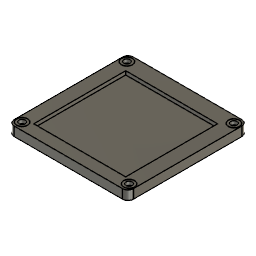
Hub_PCB_TopAndBottomCase_Assembled (Autodesk Fusion 360 archive; units mm, degrees)
design "case"
part number: 2026-03-31-19-00-49-928
Autodesk Fusion 360 part; units mm, degrees
sketch "Sketch1" plane through (0, 0, 0) normal (0, 1, 0) x (1, 0, 0)
  line L0 (0, 0) -> (50, 0)
  line L1 (50, 0) -> (50, 50)
  line L2 (50, 50) -> (0, 50)
  line L3 (0, 50) -> (0, 0)
  line L4 (-7.3367, -6.3969) -> (57.6633, -6.3969)
  line L5 (57.6633, -6.3969) -> (57.6633, 58.6031)
  line L6 (57.6633, 58.6031) -> (-7.3367, 58.6031)
  line L7 (-7.3367, 58.6031) -> (-7.3367, -6.3969)
  circle A0 centre (-3.9367, -2.3969) radius 1.7
  circle A1 centre (54.2633, -2.3969) radius 1.7
  circle A2 centre (54.2633, 54.6031) radius 1.7
  circle A3 centre (-3.9367, 54.6031) radius 1.7
  circle A4 centre (54.2633, 54.6031) radius 3
  circle A5 centre (-3.9367, 54.6031) radius 3
  circle A6 centre (-3.9367, -2.3969) radius 3
  circle A7 centre (54.2633, -2.3969) radius 3
  dimension "d3" = 65
  dimension "d4" = 65
  dimension "d5" = 3.4
  dimension "d6" = 4
  dimension "d7" = 3.4
  dimension "d8" = 3.4
  dimension "d9" = 4
  dimension "d10" = 3.4
  dimension "d11" = 3.4
  dimension "d12" = 3.4
  dimension "d13" = 4
  dimension "d14" = 3.4
  dimension "d15" = 3.4
  dimension "d16" = 4
  dimension "d17" = 6
  dimension "d18" = 6
  dimension "d19" = 6
  dimension "d20" = 6
  constraint horizontal L0
  constraint vertical L1
  constraint horizontal L2
  constraint vertical L3
  constraint coincident L0.start L3.end
  constraint horizontal L4
  constraint vertical L5
  constraint horizontal L6
  constraint vertical L7
  constraint concentric A2 A4
  constraint concentric A3 A5
  constraint concentric A0 A6
  constraint concentric A1 A7
  measures "d3" distance of L4.start L6.end
  measures "d4" distance of L5.end L6.end
  measures "d5" diameter of A0
  measures "d6" distance of L4 A0.centre
  measures "d7" distance of L7 A0.centre
  measures "d8" diameter of A1
  measures "d9" distance of L4 A1.centre
  measures "d10" distance of L5 A1.centre
  measures "d11" diameter of A2
  measures "d12" distance of L5 A2.centre
  measures "d13" distance of L6 A2.centre
  measures "d14" diameter of A3
  measures "d15" distance of L7 A3.centre
  measures "d16" distance of L6 A3.centre
  measures "d17" diameter of A4
  measures "d18" diameter of A5
  measures "d19" diameter of A6
  measures "d20" diameter of A7
extrude "Extrude1" add sketch "Sketch1" along normal blind 2 from surface at 3.1 contours A4 | A5 | A6 | A7 makes body 1 at (-0.9516, 4.4333, -54.3044) makes body 2 at (-0.9516, 4.4333, 2.6956) makes body 3 at (57.2484, 4.4333, -54.3044) makes body 4 at (57.2484, 4.4333, 2.6956)
extrude "Extrude2" add sketch "Sketch1" along normal blind 5 contours L4 L5 L6 L7 bodies 1 2 3 4
extrude "Extrude3" add sketch "Sketch1" along normal blind 3 contours L0 L1 L2 L3 bodies 1
move_body "Move1" bodies 1 to x (1, 0, 0) y (0, 0, 1) z (0, -1, 0) at (0, -58.6031, -58.6031)
fillet "Fillet1" radius 3 1 edges at (57.6633, 0, -56.1031) on bodies 1
fillet "Fillet2" radius 3 1 edges at (57.6633, -65, -56.1031) on bodies 1
fillet "Fillet3" radius 3 1 edges at (-7.3367, -65, -56.1031) on bodies 1
fillet "Fillet4" radius 3 1 edges at (-7.3367, 0, -56.1031) on bodies 1
move_body "Move2" bodies 1 to x (1, 0, 0) y (0, 1, 0) z (0, 0, 1) at (0, 0, 45)
move_body "Move3" bodies 1 to x (1, 0, 0) y (0, 1, 0) z (0, 0, 1) at (10, 0, 35)
